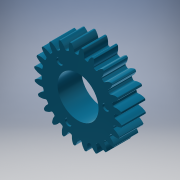
# Autodesk Inventor part: 12-0024_Gear
Saved by Autodesk Inventor 2017.1 (Build 211199000, 199)
## iProperties
Category: Gear Kit
Company: Autodesk Inc.
Created: 2014-11-29
Part Number: 12-0024_Gear
Material: Polystyrene, High Impact
Document SubType Name: Modeling
Designer: Matrix
Density: 1.022 g/cm^3
Appearance: Sky Blue Dark
Catalog Web Link: http://matrixrobotics.com/
Vendor: Matrix
Author: Autodesk Inc.
Autodesk Inventor part; units mm, degrees
ref_plane "YZ Plane" through (0, 0, 0) normal (1, 0, 0) x (0, 1, 0)
ref_plane "XZ Plane" through (0, 0, 0) normal (0, 1, 0) x (-1, 0, 0)
ref_plane "XY Plane" through (0, 0, 0) normal (0, 0, 1) x (1, 0, 0)
sketch "Sketch1" plane through (0, 0, 0) normal (0, 1, 0) x (-1, 0, 0)
  line L0 (-0.137, 10.8865) -> (-0.2406, 11.4668)
  arc A0 (-0.2406, 11.4668) -> (-0.2478, 11.4985) centre (-0.5852, 11.4053) ccw
  arc A1 (-0.2478, 11.4985) -> (-0.8281, 12.7295) centre (-4.1033, 10.4332) ccw
  arc A2 (-0.8281, 12.7295) -> (-1.0097, 12.8138) centre (-0.9919, 12.6146) ccw
  line L1 (-1.0097, 12.8138) -> (-1.2849, 12.7892)
  arc A3 (-1.2849, 12.7892) -> (-1.4486, 12.6739) centre (-1.2671, 12.59) ccw
  arc A4 (-1.4486, 12.6739) -> (-1.8008, 11.3594) centre (2.1827, 10.9966) ccw
  arc A5 (-1.8008, 11.3594) -> (-1.8022, 11.3269) centre (-1.4522, 11.3276) ccw
  line L2 (-1.8022, 11.3269) -> (-1.801, 10.7374)
  arc A6 (-2.0822, 10.3935) -> (-1.801, 10.7374) centre (-2.151, 10.7367) ccw
  arc A7 (-2.0822, 10.3935) -> (-2.549, 10.289) centre (0, 0) ccw
  arc A8 (-2.95, 10.4801) -> (-2.549, 10.289) centre (-2.6331, 10.6287) ccw
  line L3 (-2.95, 10.4801) -> (-3.2003, 11.0138)
  arc A9 (-3.2003, 11.0138) -> (-3.2154, 11.0426) centre (-3.5172, 10.8652) ccw
  arc A10 (-3.2154, 11.0426) -> (-4.0945, 12.0814) centre (-6.6638, 9.0157) ccw
  arc A11 (-4.0945, 12.0814) -> (-4.2918, 12.1159) centre (-4.223, 11.9281) ccw
  line L4 (-4.2918, 12.1159) -> (-4.5512, 12.0208)
  arc A12 (-4.5512, 12.0208) -> (-4.6794, 11.8674) centre (-4.4824, 11.8331) ccw
  arc A13 (-4.6794, 11.8674) -> (-4.6794, 10.5062) centre (-0.7378, 11.1868) ccw
  arc A14 (-4.6794, 10.5062) -> (-4.6724, 10.4745) centre (-4.3346, 10.5658) ccw
  line L5 (-4.6724, 10.4745) -> (-4.5187, 9.9054)
  arc A15 (-4.7013, 9.5004) -> (-4.5187, 9.9054) centre (-4.8565, 9.8141) ccw
  arc A16 (-4.7013, 9.5004) -> (-5.1251, 9.2787) centre (0, 0) ccw
  arc A17 (-5.5619, 9.3595) -> (-5.1251, 9.2787) centre (-5.2943, 9.585) ccw
  line L6 (-5.5619, 9.3595) -> (-5.9418, 9.8102)
  arc A18 (-5.9418, 9.8102) -> (-5.9639, 9.8341) centre (-6.2095, 9.5847) ccw
  arc A19 (-5.9639, 9.8341) -> (-7.0819, 10.61) centre (-8.7702, 6.9837) ccw
  arc A20 (-7.0819, 10.61) -> (-7.2814, 10.5922) centre (-7.1663, 10.4287) ccw
  line L7 (-7.2814, 10.5922) -> (-7.5074, 10.4333)
  arc A21 (-7.5074, 10.4333) -> (-7.5915, 10.2516) centre (-7.3923, 10.2697) ccw
  arc A22 (-7.5915, 10.2516) -> (-7.2392, 8.9371) centre (-3.608, 10.6147) ccw
  arc A23 (-7.2392, 8.9371) -> (-7.2242, 8.9082) centre (-6.9215, 9.0839) ccw
  line L8 (-7.2242, 8.9082) -> (-6.9284, 8.3984)
  arc A24 (-7, 7.9599) -> (-6.9284, 8.3984) centre (-7.2311, 8.2227) ccw
  arc A25 (-7, 7.9599) -> (-7.3519, 7.636) centre (0, 0) ccw
  arc A26 (-7.7948, 7.601) -> (-7.3519, 7.636) centre (-7.5947, 7.8882) ccw
  line L9 (-7.7948, 7.601) -> (-8.2784, 7.9381)
  arc A27 (-8.2784, 7.9381) -> (-8.3059, 7.9555) centre (-8.4786, 7.651) ccw
  arc A28 (-8.3059, 7.9555) -> (-9.5867, 8.4155) centre (-10.2789, 4.4759) ccw
  arc A29 (-9.5867, 8.4155) -> (-9.7748, 8.3468) centre (-9.6213, 8.2185) ccw
  line L10 (-9.7748, 8.3468) -> (-9.9519, 8.1348)
  arc A30 (-9.9519, 8.1348) -> (-9.9861, 7.9374) centre (-9.7984, 8.0065) ccw
  arc A31 (-9.9861, 7.9374) -> (-9.3056, 6.7589) centre (-6.2323, 9.3192) ccw
  arc A32 (-9.3056, 6.7589) -> (-9.2837, 6.7349) centre (-9.0367, 6.983) ccw
  line L11 (-9.2837, 6.7349) -> (-8.866, 6.319)
  arc A33 (-8.8217, 5.8769) -> (-8.866, 6.319) centre (-9.1129, 6.071) ccw
  arc A34 (-8.8217, 5.8769) -> (-9.0778, 5.473) centre (0, 0) ccw
  arc A35 (-9.4965, 5.3246) -> (-9.0778, 5.473) centre (-9.3775, 5.6537) ccw
  line L12 (-9.4965, 5.3246) -> (-10.0509, 5.525)
  arc A36 (-10.0509, 5.525) -> (-10.0819, 5.5346) centre (-10.1699, 5.1959) ccw
  arc A37 (-10.0819, 5.5346) -> (-11.4381, 5.6476) centre (-11.0871, 1.663) ccw
  arc A38 (-11.4381, 5.6476) -> (-11.602, 5.5325) centre (-11.4206, 5.4483) ccw
  line L13 (-11.602, 5.5325) -> (-11.7182, 5.2818)
  arc A39 (-11.7182, 5.2818) -> (-11.7002, 5.0824) centre (-11.5368, 5.1977) ccw
  arc A40 (-11.7002, 5.0824) -> (-10.7379, 4.1202) centre (-8.4319, 7.3886) ccw
  arc A41 (-10.7379, 4.1202) -> (-10.7105, 4.1027) centre (-10.5361, 4.4061) ccw
  line L14 (-10.7105, 4.1027) -> (-10.1994, 3.809)
  arc A42 (-10.0421, 3.3935) -> (-10.1994, 3.809) centre (-10.3737, 3.5055) ccw
  arc A43 (-10.0421, 3.3935) -> (-10.185, 2.937) centre (0, 0) ccw
  arc A44 (-10.551, 2.6853) -> (-10.185, 2.937) centre (-10.5213, 3.034) ccw
  line L15 (-10.551, 2.6853) -> (-11.1384, 2.7354)
  arc A45 (-11.1384, 2.7354) -> (-11.1709, 2.7367) centre (-11.1682, 2.3867) ccw
  arc A46 (-11.1709, 2.7367) -> (-12.5101, 2.4947) centre (-11.1397, -1.2632) ccw
  arc A47 (-12.5101, 2.4947) -> (-12.6386, 2.3411) centre (-12.4415, 2.3068) ccw
  line L16 (-12.686, 2.069) -> (-12.6386, 2.3411)
  arc A48 (-12.686, 2.069) -> (-12.6169, 1.881) centre (-12.4889, 2.0346) ccw
  arc A49 (-12.6169, 1.881) -> (-11.4384, 1.2006) centre (-10.0569, 4.9545) ccw
  arc A50 (-11.4384, 1.2006) -> (-11.4074, 1.1908) centre (-11.3175, 1.5291) ccw
  line L17 (-11.4074, 1.1908) -> (-10.8377, 1.0394)
  arc A51 (-10.5782, 0.6788) -> (-10.8377, 1.0394) centre (-10.9275, 0.7012) ccw
  arc A52 (-10.5782, 0.6788) -> (-10.5981, 0.2009) centre (0, 0) ccw
  arc A53 (-10.8865, -0.137) -> (-10.5981, 0.2009) centre (-10.948, 0.2075) ccw
  line L18 (-10.8865, -0.137) -> (-11.4668, -0.2406)
  arc A54 (-11.4668, -0.2406) -> (-11.4985, -0.2478) centre (-11.4053, -0.5852) ccw
  arc A55 (-11.4985, -0.2478) -> (-12.7295, -0.8281) centre (-10.4332, -4.1033) ccw
  arc A56 (-12.7295, -0.8281) -> (-12.8138, -1.0097) centre (-12.6146, -0.9919) ccw
  line L19 (-12.8138, -1.0097) -> (-12.7892, -1.2849)
  arc A57 (-12.7892, -1.2849) -> (-12.6739, -1.4486) centre (-12.59, -1.2671) ccw
  arc A58 (-12.6739, -1.4486) -> (-11.3594, -1.8008) centre (-10.9966, 2.1827) ccw
  arc A59 (-11.3594, -1.8008) -> (-11.3269, -1.8022) centre (-11.3276, -1.4522) ccw
  line L20 (-11.3269, -1.8022) -> (-10.7374, -1.801)
  arc A60 (-10.3935, -2.0822) -> (-10.7374, -1.801) centre (-10.7367, -2.151) ccw
  arc A61 (-10.3935, -2.0822) -> (-10.289, -2.549) centre (0, 0) ccw
  arc A62 (-10.4801, -2.95) -> (-10.289, -2.549) centre (-10.6287, -2.6331) ccw
  line L21 (-10.4801, -2.95) -> (-11.0138, -3.2003)
  arc A63 (-11.0138, -3.2003) -> (-11.0426, -3.2154) centre (-10.8652, -3.5172) ccw
  arc A64 (-11.0426, -3.2154) -> (-12.0814, -4.0945) centre (-9.0157, -6.6638) ccw
  arc A65 (-12.0814, -4.0945) -> (-12.1159, -4.2918) centre (-11.9281, -4.223) ccw
  line L22 (-12.1159, -4.2918) -> (-12.0208, -4.5512)
  arc A66 (-12.0208, -4.5512) -> (-11.8671, -4.6795) centre (-11.8331, -4.4824) ccw
  arc A67 (-11.8671, -4.6795) -> (-10.5062, -4.6794) centre (-11.1868, -0.7378) ccw
  arc A68 (-10.5062, -4.6794) -> (-10.4745, -4.6724) centre (-10.5658, -4.3346) ccw
  line L23 (-10.4745, -4.6724) -> (-9.9054, -4.5187)
  arc A69 (-9.5004, -4.7013) -> (-9.9054, -4.5187) centre (-9.8141, -4.8565) ccw
  arc A70 (-9.5004, -4.7013) -> (-9.2787, -5.1251) centre (0, 0) ccw
  arc A71 (-9.3595, -5.5619) -> (-9.2787, -5.1251) centre (-9.585, -5.2943) ccw
  line L24 (-9.3595, -5.5619) -> (-9.8102, -5.9418)
  arc A72 (-9.8102, -5.9418) -> (-9.8341, -5.9639) centre (-9.5847, -6.2095) ccw
  arc A73 (-9.8341, -5.9639) -> (-10.61, -7.0819) centre (-6.9837, -8.7702) ccw
  arc A74 (-10.61, -7.0819) -> (-10.5922, -7.2814) centre (-10.4287, -7.1663) ccw
  line L25 (-10.5922, -7.2814) -> (-10.4333, -7.5074)
  arc A75 (-10.4333, -7.5074) -> (-10.2516, -7.5915) centre (-10.2697, -7.3923) ccw
  arc A76 (-10.2516, -7.5915) -> (-8.9371, -7.2392) centre (-10.6147, -3.608) ccw
  arc A77 (-8.9371, -7.2392) -> (-8.9082, -7.2242) centre (-9.0839, -6.9215) ccw
  line L26 (-8.9082, -7.2242) -> (-8.3984, -6.9284)
  arc A78 (-7.9599, -7) -> (-8.3984, -6.9284) centre (-8.2227, -7.2311) ccw
  arc A79 (-7.9599, -7) -> (-7.636, -7.3519) centre (0, 0) ccw
  arc A80 (-7.601, -7.7948) -> (-7.636, -7.3519) centre (-7.8882, -7.5947) ccw
  line L27 (-7.601, -7.7948) -> (-7.9381, -8.2784)
  arc A81 (-7.9381, -8.2784) -> (-7.9555, -8.3059) centre (-7.651, -8.4786) ccw
  arc A82 (-7.9555, -8.3059) -> (-8.4155, -9.5867) centre (-4.4759, -10.2789) ccw
  arc A83 (-8.4155, -9.5867) -> (-8.3468, -9.7748) centre (-8.2185, -9.6213) ccw
  line L28 (-8.3468, -9.7748) -> (-8.1348, -9.9519)
  arc A84 (-8.1348, -9.9519) -> (-7.9374, -9.9861) centre (-8.0065, -9.7984) ccw
  arc A85 (-7.9374, -9.9861) -> (-6.7589, -9.3056) centre (-9.3192, -6.2323) ccw
  arc A86 (-6.7589, -9.3056) -> (-6.7349, -9.2837) centre (-6.983, -9.0367) ccw
  line L29 (-6.7349, -9.2837) -> (-6.319, -8.866)
  arc A87 (-5.8769, -8.8217) -> (-6.319, -8.866) centre (-6.071, -9.1129) ccw
  arc A88 (-5.8769, -8.8217) -> (-5.473, -9.0778) centre (0, 0) ccw
  arc A89 (-5.3246, -9.4965) -> (-5.473, -9.0778) centre (-5.6537, -9.3775) ccw
  line L30 (-5.3246, -9.4965) -> (-5.525, -10.0509)
  arc A90 (-5.525, -10.0509) -> (-5.5346, -10.0819) centre (-5.1959, -10.1699) ccw
  arc A91 (-5.5346, -10.0819) -> (-5.6476, -11.4381) centre (-1.663, -11.0871) ccw
  arc A92 (-5.6476, -11.4381) -> (-5.5325, -11.602) centre (-5.4483, -11.4206) ccw
  line L31 (-5.5325, -11.602) -> (-5.2818, -11.7182)
  arc A93 (-5.2818, -11.7182) -> (-5.0824, -11.7002) centre (-5.1977, -11.5368) ccw
  arc A94 (-5.0824, -11.7002) -> (-4.1202, -10.7379) centre (-7.3886, -8.4319) ccw
  arc A95 (-4.1202, -10.7379) -> (-4.1027, -10.7105) centre (-4.4061, -10.5361) ccw
  line L32 (-4.1027, -10.7105) -> (-3.809, -10.1994)
  arc A96 (-3.3935, -10.0421) -> (-3.809, -10.1994) centre (-3.5055, -10.3737) ccw
  arc A97 (-3.3935, -10.0421) -> (-2.937, -10.185) centre (0, 0) ccw
  arc A98 (-2.6853, -10.551) -> (-2.937, -10.185) centre (-3.034, -10.5213) ccw
  line L33 (-2.6853, -10.551) -> (-2.7354, -11.1384)
  arc A99 (-2.7354, -11.1384) -> (-2.7367, -11.1709) centre (-2.3867, -11.1682) ccw
  arc A100 (-2.7367, -11.1709) -> (-2.4947, -12.5101) centre (1.2632, -11.1397) ccw
  arc A101 (-2.4947, -12.5101) -> (-2.3411, -12.6386) centre (-2.3068, -12.4415) ccw
  line L34 (-2.069, -12.686) -> (-2.3411, -12.6386)
  arc A102 (-2.069, -12.686) -> (-1.881, -12.6169) centre (-2.0346, -12.4889) ccw
  arc A103 (-1.881, -12.6169) -> (-1.2006, -11.4384) centre (-4.9545, -10.0569) ccw
  arc A104 (-1.2006, -11.4384) -> (-1.1908, -11.4074) centre (-1.5291, -11.3175) ccw
  line L35 (-1.1908, -11.4074) -> (-1.0394, -10.8377)
  arc A105 (-0.6788, -10.5782) -> (-1.0394, -10.8377) centre (-0.7012, -10.9275) ccw
  arc A106 (-0.6788, -10.5782) -> (-0.2009, -10.5981) centre (0, 0) ccw
  arc A107 (0.137, -10.8865) -> (-0.2009, -10.5981) centre (-0.2075, -10.948) ccw
  line L36 (0.137, -10.8865) -> (0.2406, -11.4668)
  arc A108 (0.2406, -11.4668) -> (0.2478, -11.4985) centre (0.5852, -11.4053) ccw
  arc A109 (0.2478, -11.4985) -> (0.8281, -12.7295) centre (4.1033, -10.4332) ccw
  arc A110 (0.8281, -12.7295) -> (1.0097, -12.8138) centre (0.9919, -12.6146) ccw
  line L37 (1.0097, -12.8138) -> (1.2849, -12.7892)
  arc A111 (1.2849, -12.7892) -> (1.4486, -12.6739) centre (1.2671, -12.59) ccw
  arc A112 (1.4486, -12.6739) -> (1.8008, -11.3594) centre (-2.1827, -10.9966) ccw
  arc A113 (1.8008, -11.3594) -> (1.8022, -11.3269) centre (1.4522, -11.3276) ccw
  line L38 (1.8022, -11.3269) -> (1.801, -10.7374)
  arc A114 (2.0822, -10.3935) -> (1.801, -10.7374) centre (2.151, -10.7367) ccw
  arc A115 (2.0822, -10.3935) -> (2.549, -10.289) centre (0, 0) ccw
  arc A116 (2.95, -10.4801) -> (2.549, -10.289) centre (2.6331, -10.6287) ccw
  line L39 (2.95, -10.4801) -> (3.2003, -11.0138)
  arc A117 (3.2003, -11.0138) -> (3.2154, -11.0426) centre (3.5172, -10.8652) ccw
  arc A118 (3.2154, -11.0426) -> (4.0945, -12.0814) centre (6.6638, -9.0157) ccw
  arc A119 (4.0945, -12.0814) -> (4.2918, -12.1159) centre (4.223, -11.9281) ccw
  line L40 (4.2918, -12.1159) -> (4.5512, -12.0208)
  arc A120 (4.5512, -12.0208) -> (4.6795, -11.8671) centre (4.4824, -11.8331) ccw
  arc A121 (4.6795, -11.8671) -> (4.6794, -10.5062) centre (0.7378, -11.1868) ccw
  arc A122 (4.6794, -10.5062) -> (4.6724, -10.4745) centre (4.3346, -10.5658) ccw
  line L41 (4.6724, -10.4745) -> (4.5187, -9.9054)
  arc A123 (4.7013, -9.5004) -> (4.5187, -9.9054) centre (4.8565, -9.8141) ccw
  arc A124 (4.7013, -9.5004) -> (5.1251, -9.2787) centre (0, 0) ccw
  arc A125 (5.5619, -9.3595) -> (5.1251, -9.2787) centre (5.2943, -9.585) ccw
  line L42 (5.5619, -9.3595) -> (5.9418, -9.8102)
  arc A126 (5.9418, -9.8102) -> (5.9639, -9.8341) centre (6.2095, -9.5847) ccw
  arc A127 (5.9639, -9.8341) -> (7.0819, -10.61) centre (8.7702, -6.9837) ccw
  arc A128 (7.0819, -10.61) -> (7.2814, -10.5922) centre (7.1663, -10.4287) ccw
  line L43 (7.2814, -10.5922) -> (7.5074, -10.4333)
  arc A129 (7.5074, -10.4333) -> (7.5915, -10.2516) centre (7.3923, -10.2697) ccw
  arc A130 (7.5915, -10.2516) -> (7.2392, -8.9371) centre (3.608, -10.6147) ccw
  arc A131 (7.2392, -8.9371) -> (7.2242, -8.9082) centre (6.9215, -9.0839) ccw
  line L44 (7.2242, -8.9082) -> (6.9284, -8.3984)
  arc A132 (7, -7.9599) -> (6.9284, -8.3984) centre (7.2311, -8.2227) ccw
  arc A133 (7, -7.9599) -> (7.3519, -7.636) centre (0, 0) ccw
  arc A134 (7.7948, -7.601) -> (7.3519, -7.636) centre (7.5947, -7.8882) ccw
  line L45 (7.7948, -7.601) -> (8.2784, -7.9381)
  arc A135 (8.2784, -7.9381) -> (8.3059, -7.9555) centre (8.4786, -7.651) ccw
  arc A136 (8.3059, -7.9555) -> (9.5867, -8.4155) centre (10.2789, -4.4759) ccw
  arc A137 (9.5867, -8.4155) -> (9.7748, -8.3468) centre (9.6213, -8.2185) ccw
  line L46 (9.7748, -8.3468) -> (9.9519, -8.1348)
  arc A138 (9.9519, -8.1348) -> (9.9861, -7.9374) centre (9.7984, -8.0065) ccw
  arc A139 (9.9861, -7.9374) -> (9.3056, -6.7589) centre (6.2323, -9.3192) ccw
  arc A140 (9.3056, -6.7589) -> (9.2837, -6.7349) centre (9.0367, -6.983) ccw
  line L47 (9.2837, -6.7349) -> (8.866, -6.319)
  arc A141 (8.8217, -5.8769) -> (8.866, -6.319) centre (9.1129, -6.071) ccw
  arc A142 (8.8217, -5.8769) -> (9.0778, -5.473) centre (0, 0) ccw
  arc A143 (9.4965, -5.3246) -> (9.0778, -5.473) centre (9.3775, -5.6537) ccw
  line L48 (9.4965, -5.3246) -> (10.0509, -5.525)
  arc A144 (10.0509, -5.525) -> (10.0819, -5.5346) centre (10.1699, -5.1959) ccw
  arc A145 (10.0819, -5.5346) -> (11.4381, -5.6476) centre (11.0871, -1.663) ccw
  arc A146 (11.4381, -5.6476) -> (11.602, -5.5325) centre (11.4206, -5.4483) ccw
  line L49 (11.602, -5.5325) -> (11.7182, -5.2818)
  arc A147 (11.7182, -5.2818) -> (11.7002, -5.0824) centre (11.5368, -5.1977) ccw
  arc A148 (11.7002, -5.0824) -> (10.7379, -4.1202) centre (8.4319, -7.3886) ccw
  arc A149 (10.7379, -4.1202) -> (10.7105, -4.1027) centre (10.5361, -4.4061) ccw
  line L50 (10.7105, -4.1027) -> (10.1994, -3.809)
  arc A150 (10.0421, -3.3935) -> (10.1994, -3.809) centre (10.3737, -3.5055) ccw
  arc A151 (10.0421, -3.3935) -> (10.185, -2.937) centre (0, 0) ccw
  arc A152 (10.551, -2.6853) -> (10.185, -2.937) centre (10.5213, -3.034) ccw
  line L51 (10.551, -2.6853) -> (11.1384, -2.7354)
  arc A153 (11.1384, -2.7354) -> (11.1709, -2.7367) centre (11.1682, -2.3867) ccw
  arc A154 (11.1709, -2.7367) -> (12.5101, -2.4947) centre (11.1397, 1.2632) ccw
  arc A155 (12.5101, -2.4947) -> (12.6386, -2.3411) centre (12.4415, -2.3068) ccw
  line L52 (12.686, -2.069) -> (12.6386, -2.3411)
  arc A156 (12.686, -2.069) -> (12.6169, -1.881) centre (12.4889, -2.0346) ccw
  arc A157 (12.6169, -1.881) -> (11.4384, -1.2006) centre (10.0569, -4.9545) ccw
  arc A158 (11.4384, -1.2006) -> (11.4074, -1.1908) centre (11.3175, -1.5291) ccw
  line L53 (11.4074, -1.1908) -> (10.8377, -1.0394)
  arc A159 (10.5782, -0.6788) -> (10.8377, -1.0394) centre (10.9275, -0.7012) ccw
  arc A160 (10.5782, -0.6788) -> (10.5981, -0.2009) centre (0, 0) ccw
  arc A161 (10.8865, 0.137) -> (10.5981, -0.2009) centre (10.948, -0.2075) ccw
  line L54 (10.8865, 0.137) -> (11.4668, 0.2406)
  arc A162 (11.4668, 0.2406) -> (11.4985, 0.2478) centre (11.4053, 0.5852) ccw
  arc A163 (11.4985, 0.2478) -> (12.7295, 0.8281) centre (10.4332, 4.1033) ccw
  arc A164 (12.7295, 0.8281) -> (12.8138, 1.0097) centre (12.6146, 0.9919) ccw
  line L55 (12.8138, 1.0097) -> (12.7892, 1.2849)
  arc A165 (12.7892, 1.2849) -> (12.6739, 1.4486) centre (12.59, 1.2671) ccw
  arc A166 (12.6739, 1.4486) -> (11.3594, 1.8008) centre (10.9966, -2.1827) ccw
  arc A167 (11.3594, 1.8008) -> (11.3269, 1.8022) centre (11.3276, 1.4522) ccw
  line L56 (11.3269, 1.8022) -> (10.7374, 1.801)
  arc A168 (10.3935, 2.0822) -> (10.7374, 1.801) centre (10.7367, 2.151) ccw
  arc A169 (10.3935, 2.0822) -> (10.289, 2.549) centre (0, 0) ccw
  arc A170 (10.4801, 2.95) -> (10.289, 2.549) centre (10.6287, 2.6331) ccw
  line L57 (10.4801, 2.95) -> (11.0138, 3.2003)
  arc A171 (11.0138, 3.2003) -> (11.0426, 3.2154) centre (10.8652, 3.5172) ccw
  arc A172 (11.0426, 3.2154) -> (12.0814, 4.0945) centre (9.0157, 6.6638) ccw
  arc A173 (12.0814, 4.0945) -> (12.1159, 4.2918) centre (11.9281, 4.223) ccw
  line L58 (12.1159, 4.2918) -> (12.0208, 4.5512)
  arc A174 (12.0208, 4.5512) -> (11.8671, 4.6795) centre (11.8331, 4.4824) ccw
  arc A175 (11.8671, 4.6795) -> (10.5062, 4.6794) centre (11.1868, 0.7378) ccw
  arc A176 (10.5062, 4.6794) -> (10.4745, 4.6724) centre (10.5658, 4.3346) ccw
  line L59 (10.4745, 4.6724) -> (9.9054, 4.5187)
  arc A177 (9.5004, 4.7013) -> (9.9054, 4.5187) centre (9.8141, 4.8565) ccw
  arc A178 (9.5004, 4.7013) -> (9.2787, 5.1251) centre (0, 0) ccw
  arc A179 (9.3595, 5.5619) -> (9.2787, 5.1251) centre (9.585, 5.2943) ccw
  line L60 (9.3595, 5.5619) -> (9.8102, 5.9418)
  arc A180 (9.8102, 5.9418) -> (9.8341, 5.9639) centre (9.5847, 6.2095) ccw
  arc A181 (9.8341, 5.9639) -> (10.61, 7.0819) centre (6.9837, 8.7702) ccw
  arc A182 (10.61, 7.0819) -> (10.5922, 7.2814) centre (10.4287, 7.1663) ccw
  line L61 (10.5922, 7.2814) -> (10.4333, 7.5074)
  arc A183 (10.4333, 7.5074) -> (10.2516, 7.5915) centre (10.2697, 7.3923) ccw
  arc A184 (10.2516, 7.5915) -> (8.9371, 7.2392) centre (10.6147, 3.608) ccw
  arc A185 (8.9371, 7.2392) -> (8.9082, 7.2242) centre (9.0839, 6.9215) ccw
  line L62 (8.9082, 7.2242) -> (8.3984, 6.9284)
  arc A186 (7.9599, 7) -> (8.3984, 6.9284) centre (8.2227, 7.2311) ccw
  arc A187 (7.9599, 7) -> (7.636, 7.3519) centre (0, 0) ccw
  arc A188 (7.601, 7.7948) -> (7.636, 7.3519) centre (7.8882, 7.5947) ccw
  line L63 (7.601, 7.7948) -> (7.9381, 8.2784)
  arc A189 (7.9381, 8.2784) -> (7.9555, 8.3059) centre (7.651, 8.4786) ccw
  arc A190 (7.9555, 8.3059) -> (8.4155, 9.5867) centre (4.4759, 10.2789) ccw
  arc A191 (8.4155, 9.5867) -> (8.3468, 9.7748) centre (8.2185, 9.6213) ccw
  line L64 (8.3468, 9.7748) -> (8.1348, 9.9519)
  arc A192 (8.1348, 9.9519) -> (7.9374, 9.9861) centre (8.0065, 9.7984) ccw
  arc A193 (7.9374, 9.9861) -> (6.7589, 9.3056) centre (9.3192, 6.2323) ccw
  arc A194 (6.7589, 9.3056) -> (6.7349, 9.2837) centre (6.983, 9.0367) ccw
  line L65 (6.7349, 9.2837) -> (6.319, 8.866)
  arc A195 (5.8769, 8.8217) -> (6.319, 8.866) centre (6.071, 9.1129) ccw
  arc A196 (5.8769, 8.8217) -> (5.473, 9.0778) centre (0, 0) ccw
  arc A197 (5.3246, 9.4965) -> (5.473, 9.0778) centre (5.6537, 9.3775) ccw
  line L66 (5.3246, 9.4965) -> (5.525, 10.0509)
  arc A198 (5.525, 10.0509) -> (5.5346, 10.0819) centre (5.1959, 10.1699) ccw
  arc A199 (5.5346, 10.0819) -> (5.6476, 11.4381) centre (1.663, 11.0871) ccw
  arc A200 (5.6476, 11.4381) -> (5.5325, 11.602) centre (5.4483, 11.4206) ccw
  line L67 (5.5325, 11.602) -> (5.2818, 11.7182)
  arc A201 (5.2818, 11.7182) -> (5.0824, 11.7002) centre (5.1977, 11.5368) ccw
  arc A202 (5.0824, 11.7002) -> (4.1202, 10.7379) centre (7.3886, 8.4319) ccw
  arc A203 (4.1202, 10.7379) -> (4.1027, 10.7105) centre (4.4061, 10.5361) ccw
  line L68 (4.1027, 10.7105) -> (3.809, 10.1994)
  arc A204 (3.3935, 10.0421) -> (3.809, 10.1994) centre (3.5055, 10.3737) ccw
  arc A205 (3.3935, 10.0421) -> (2.937, 10.185) centre (0, 0) ccw
  arc A206 (2.6853, 10.551) -> (2.937, 10.185) centre (3.034, 10.5213) ccw
  line L69 (2.6853, 10.551) -> (2.7354, 11.1384)
  arc A207 (2.7354, 11.1384) -> (2.7367, 11.1709) centre (2.3867, 11.1682) ccw
  arc A208 (2.7367, 11.1709) -> (2.4947, 12.5101) centre (-1.2632, 11.1397) ccw
  arc A209 (2.4947, 12.5101) -> (2.3411, 12.6386) centre (2.3068, 12.4415) ccw
  line L70 (2.069, 12.686) -> (2.3411, 12.6386)
  arc A210 (2.069, 12.686) -> (1.881, 12.6169) centre (2.0346, 12.4889) ccw
  arc A211 (1.881, 12.6169) -> (1.2006, 11.4384) centre (4.9545, 10.0569) ccw
  arc A212 (1.2006, 11.4384) -> (1.1908, 11.4074) centre (1.5291, 11.3175) ccw
  line L71 (1.1908, 11.4074) -> (1.0394, 10.8377)
  arc A213 (0.6788, 10.5782) -> (1.0394, 10.8377) centre (0.7012, 10.9275) ccw
  arc A214 (0.6788, 10.5782) -> (0.2009, 10.5981) centre (0, 0) ccw
  arc A215 (-0.137, 10.8865) -> (0.2009, 10.5981) centre (0.2075, 10.948) ccw
  circle A216 centre (0, 0) radius 6
  point P0 (0, 0)
  point P1 (0, 0)
  constraints: 432 point on circle, 217 centre point, 144 end point
extrude "Extrusion1" add sketch "Sketch1" against normal blind 7
sketch "Sketch2" plane through (0, -7, 0) normal (0, -1, 0) x (1, 0, 0)
  circle A0 centre (8.1709, 1.458) radius 1
  circle A1 centre (-2.8228, -7.8052) radius 1
  circle A2 centre (-5.3481, 6.3473) radius 1
  point P0 (0, 0)
  point P1 (0, 0)
  point P2 (0, 0)
  constraints: 3 centre point
extrude "Extrusion2" cut sketch "Sketch2" against normal blind 0.5
body "Solid1"
